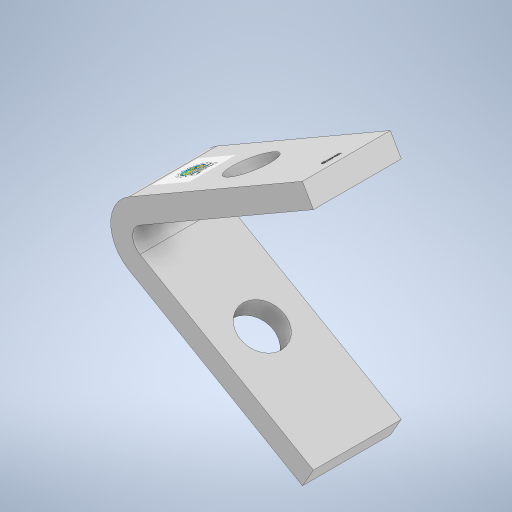
# Autodesk Inventor part: Part1
Saved by Autodesk Inventor 2023 (Build 270158000, 158)
## iProperties
Created: 2024-10-14
Part Number: Part1
Material: Generic
Document SubType Name: Modeling
Designer: students
Density: 1 g/cm^3
Appearance: Default
Author: students
Autodesk Inventor part; units mm, degrees
ref_plane "YZ Plane" through (0, 0, 0) normal (1, 0, 0) x (0, 1, 0)
ref_plane "XZ Plane" through (0, 0, 0) normal (0, 1, 0) x (-1, 0, 0)
ref_plane "XY Plane" through (0, 0, 0) normal (0, 0, 1) x (1, 0, 0)
sketch "Sketch1" plane through (0, 0, 0) normal (0, 0, 1) x (1, 0, 0)
  line L0 (57.8268, 26.3393) -> (176.2114, 94.6887)
  line L1 (20.3268, 4.6887) -> (157.0255, 4.6887) construction
  line L2 (57.8268, -16.9619) -> (176.2114, -85.3113)
  line L3 (20.3268, 4.6887) -> (157.0255, 4.6887) construction
  arc A0 (57.8268, 26.3393) -> (57.8268, -16.9619) centre (70.3268, 4.6887) ccw
  line L4 (183.7114, 81.6983) -> (65.3268, 13.3489)
  arc A1 (65.3268, 13.3489) -> (65.3268, -3.9716) centre (70.3268, 4.6887) ccw
  line L5 (65.3268, -3.9716) -> (183.7114, -72.3209)
  line L6 (176.2114, 94.6887) -> (183.7114, 81.6983)
  line L7 (183.7114, -72.3209) -> (176.2114, -85.3113)
  point P0 (0, 0)
  dimension "d0" = 180
  dimension "d2" = 180
  dimension "d4" = 25
  dimension "d5" = 15
  dimension "d7" = 60
  constraints: 16 end point, 4 point on circle, 2 centre point, 2 equal length, 2 horizontal, 2 point on line, 2 tangent, 2 other
  measures "d0" distance of L1.start L0.end
  measures "d2" distance of L1.start L2.end
  measures "d4" radius of A0
  measures "d5" distance between parallel lines of L0 L4
  measures "d7" angle of L5 L4
extrude "Extrusion1" add sketch "Sketch1" along normal blind 60
sketch "Sketch2" plane through (57.8268, 26.3393, 60) normal (-0.5, 0.8660254, 0) x (0.8660254, 0.5, 0)
  line L0 (136.6987, 60) -> (136.6987, 0) projected
  line L1 (136.6987, 60) -> (136.6987, 30)
  circle A0 centre (61.6987, 30) radius 15
  point P0 (-63.2492, 60)
  dimension "d10" = 30
  dimension "d12" = 30
  constraints: 2 end point, 1 centre point, 1 midpoint
  measures "d10" distance of L0.start L1.end
  measures "d12" diameter of A0
hole "Hole1" at (111.2595, 57.1887, 30) direction (0.5, -0.8660254, 0) diameter 30 depth 16 tip angle 118
sketch "Sketch3" plane through (176.2114, -85.3113, 0) normal (-0.5, -0.8660254, 0) x (0.8660254, -0.5, 0)
  line L0 (0, 60) -> (0, 30)
  line L1 (0, 0) -> (0, 60) projected
  line L2 (0, 30) -> (-75, 30)
  circle A0 centre (-75, 30) radius 15
  point P0 (-195.2592, 0)
  dimension "d20" = 30
  dimension "d21" = 75
  dimension "d22" = 30
  constraints: 4 end point, 1 centre point, 1 coincident, 1 midpoint, 1 perpendicular
  measures "d20" distance of L0.start L0.end
  measures "d21" distance of L0.end L2.end
  measures "d22" diameter of A0
hole "Hole2" at (111.2595, -47.8113, 30) direction (0.5, 0.8660254, 0) diameter 30 depth 16 tip angle 118
sketch "Sketch8" plane through (57.8268, 26.3393, 60) normal (-0.5, 0.8660254, 0) x (0.8660254, 0.5, 0)
  line L0 (124.5742, 21.8974) -> (124.5742, 35.2858) construction
  line L1 (124.5742, 35.2858) -> (128.6544, 35.2858) construction
  line L2 (128.6544, 35.2858) -> (128.6544, 21.8974) construction
  line L3 (128.6544, 21.8974) -> (124.5742, 21.8974) construction
  line L4 (0, 60) -> (0, 0) projected
  line L5 (0, 27.6079) -> (153.6173, 28.7907) construction
  line L6 (127.758, 23.9352) -> (127.758, 23.5499)
  line L7 (127.758, 23.5499) -> (127.5258, 23.5499)
  spline S0 degree 2 poles (127.5258, 23.5499) (127.5999, 23.461) (127.6987, 23.33) (127.7407, 23.2411) knots 0 0 0 1 2 2 2
  spline S1 degree 2 poles (127.7407, 23.2411) (127.7803, 23.1596) (127.8222, 22.9842) (127.8222, 22.8681) knots 0 0 0 1 2 2 2
  spline S2 degree 2 poles (127.8222, 22.8681) (127.8222, 22.6804) (127.6666, 22.3643) (127.516, 22.2531) knots 0 0 0 1 2 2 2
  spline S3 degree 2 poles (127.516, 22.2531) (127.3653, 22.142) (126.9207, 22.0185) (126.6317, 22.0185) knots 0 0 0 1 2 2 2
  spline S4 degree 2 poles (126.6317, 22.0185) (126.3304, 22.0185) (125.8907, 22.1741) (125.7252, 22.3099) knots 0 0 0 1 2 2 2
  spline S5 degree 2 poles (125.7252, 22.3099) (125.577, 22.4359) (125.4066, 22.7891) (125.4066, 22.9842) knots 0 0 0 1 2 2 2
  spline S6 degree 2 poles (125.4066, 22.9842) (125.4066, 23.1547) (125.4831, 23.4091) (125.5622, 23.5499) knots 0 0 0 1 2 2 2
  line L8 (125.5622, 23.5499) -> (124.5742, 23.5499)
  line L9 (124.5742, 23.5499) -> (124.5742, 23.9352)
  line L10 (124.5742, 23.9352) -> (127.758, 23.9352)
  line L11 (127.2023, 23.5499) -> (125.8808, 23.5499)
  spline S7 degree 2 poles (125.8808, 23.5499) (125.8117, 23.4066) (125.7598, 23.1794) (125.7598, 23.0485) knots 0 0 0 1 2 2 2
  spline S8 degree 2 poles (125.7598, 23.0485) (125.7598, 22.7521) (126.2044, 22.4161) (126.6243, 22.4161) knots 0 0 0 1 2 2 2
  spline S9 degree 2 poles (126.6243, 22.4161) (127.0294, 22.4161) (127.4567, 22.673) (127.4567, 22.9571) knots 0 0 0 1 2 2 2
  spline S10 degree 2 poles (127.4567, 22.9571) (127.4567, 23.1077) (127.3184, 23.414) (127.2023, 23.5499) knots 0 0 0 1 2 2 2
  line L12 (127.758, 26.2891) -> (127.758, 25.9038)
  line L13 (127.758, 25.9038) -> (126.4539, 25.9038)
  spline S11 degree 2 poles (126.4539, 25.9038) (126.2958, 25.9038) (126.0241, 25.8742) (125.9426, 25.8297) knots 0 0 0 1 2 2 2
  spline S12 degree 2 poles (125.9426, 25.8297) (125.8561, 25.7828) (125.7721, 25.6148) (125.7721, 25.4715) knots 0 0 0 1 2 2 2
  spline S13 degree 2 poles (125.7721, 25.4715) (125.7721, 25.3283) (125.9253, 25.0245) (126.0488, 24.8787) knots 0 0 0 1 2 2 2
  line L14 (126.0488, 24.8787) -> (127.758, 24.8787)
  line L15 (127.758, 24.8787) -> (127.758, 24.4934)
  line L16 (127.758, 24.4934) -> (124.5742, 24.4934)
  line L17 (124.5742, 24.4934) -> (124.5742, 24.8787)
  line L18 (124.5742, 24.8787) -> (125.7252, 24.8787)
  spline S14 degree 2 poles (125.7252, 24.8787) (125.5696, 25.0516) (125.4066, 25.3851) (125.4066, 25.5728) knots 0 0 0 1 2 2 2
  spline S15 degree 2 poles (125.4066, 25.5728) (125.4066, 25.9087) (125.8512, 26.2891) (126.2735, 26.2891) knots 0 0 0 1 2 2 2
  line L19 (126.2735, 26.2891) -> (127.758, 26.2891)
  spline S16 degree 2 poles (127.516, 28.1046) (127.5505, 28.0577) (127.674, 27.8996) (127.7111, 27.8255) knots 0 0 0 1 2 2 2
  spline S17 degree 2 poles (127.7111, 27.8255) (127.7654, 27.7242) (127.8222, 27.534) (127.8222, 27.3611) knots 0 0 0 1 2 2 2
  spline S18 degree 2 poles (127.8222, 27.3611) (127.8222, 27.2203) (127.716, 26.9659) (127.6197, 26.8696) knots 0 0 0 1 2 2 2
  spline S19 degree 2 poles (127.6197, 26.8696) (127.5258, 26.7782) (127.2492, 26.667) (127.0961, 26.667) knots 0 0 0 1 2 2 2
  spline S20 degree 2 poles (127.0961, 26.667) (126.8589, 26.667) (126.523, 26.8671) (126.4267, 27.0845) knots 0 0 0 1 2 2 2
  spline S21 degree 2 poles (126.4267, 27.0845) (126.3378, 27.2771) (126.2711, 27.8008) (126.2538, 28.1046) knots 0 0 0 1 2 2 2
  line L20 (126.2538, 28.1046) -> (126.1797, 28.1046)
  spline S22 degree 2 poles (126.1797, 28.1046) (126.0463, 28.1046) (125.8808, 28.0231) (125.8339, 27.949) knots 0 0 0 1 2 2 2
  spline S23 degree 2 poles (125.8339, 27.949) (125.787, 27.8749) (125.7573, 27.6624) (125.7573, 27.5488) knots 0 0 0 1 2 2 2
  spline S24 degree 2 poles (125.7573, 27.5488) (125.7573, 27.4154) (125.8364, 27.0548) (125.9129, 26.8745) knots 0 0 0 1 2 2 2
  line L21 (125.9129, 26.8745) -> (125.9129, 26.8523)
  line L22 (125.9129, 26.8523) -> (125.5202, 26.8523)
  spline S25 degree 2 poles (125.5202, 26.8523) (125.4905, 26.9585) (125.4164, 27.3562) (125.4164, 27.5513) knots 0 0 0 1 2 2 2
  spline S26 degree 2 poles (125.4164, 27.5513) (125.4164, 27.7884) (125.4905, 28.112) (125.5869, 28.2404) knots 0 0 0 1 2 2 2
  spline S27 degree 2 poles (125.5869, 28.2404) (125.6807, 28.3664) (125.9796, 28.4899) (126.1945, 28.4899) knots 0 0 0 1 2 2 2
  line L23 (126.1945, 28.4899) -> (127.758, 28.4899)
  line L24 (127.758, 28.4899) -> (127.758, 28.1046)
  line L25 (127.758, 28.1046) -> (127.516, 28.1046)
  line L26 (127.1949, 28.1046) -> (126.5601, 28.1046)
  spline S28 degree 2 poles (126.5601, 28.1046) (126.5724, 27.9663) (126.6144, 27.5488) (126.6539, 27.4179) knots 0 0 0 1 2 2 2
  spline S29 degree 2 poles (126.6539, 27.4179) (126.7009, 27.2648) (126.896, 27.0647) (127.0689, 27.0647) knots 0 0 0 1 2 2 2
  spline S30 degree 2 poles (127.0689, 27.0647) (127.2665, 27.0647) (127.4666, 27.287) (127.4666, 27.4994) knots 0 0 0 1 2 2 2
  spline S31 degree 2 poles (127.4666, 27.4994) (127.4666, 27.6797) (127.311, 27.9761) (127.1949, 28.1046) knots 0 0 0 1 2 2 2
  line L27 (125.8833, 30.2436) -> (125.8833, 30.2239)
  spline S32 degree 2 poles (125.8833, 30.2239) (125.8709, 30.1794) (125.866, 30.0831) (125.866, 30.0164) knots 0 0 0 1 2 2 2
  spline S33 degree 2 poles (125.866, 30.0164) (125.866, 29.8608) (126.0018, 29.5545) (126.1352, 29.4162) knots 0 0 0 1 2 2 2
  line L28 (126.1352, 29.4162) -> (127.758, 29.4162)
  line L29 (127.758, 29.4162) -> (127.758, 29.0308)
  line L30 (127.758, 29.0308) -> (125.4708, 29.0308)
  line L31 (125.4708, 29.0308) -> (125.4708, 29.4162)
  line L32 (125.4708, 29.4162) -> (125.8117, 29.4162)
  spline S34 degree 2 poles (125.8117, 29.4162) (125.6239, 29.6261) (125.4708, 29.9398) (125.4708, 30.088) knots 0 0 0 1 2 2 2
  spline S35 degree 2 poles (125.4708, 30.088) (125.4708, 30.1473) (125.4757, 30.2066) (125.4831, 30.2436) knots 0 0 0 1 2 2 2
  line L33 (125.4831, 30.2436) -> (125.8833, 30.2436)
  spline S36 degree 2 poles (127.8099, 31.5354) (127.8099, 30.9871) (127.1949, 30.3844) (126.6268, 30.3844) knots 0 0 0 1 2 2 2
  spline S37 degree 2 poles (126.6268, 30.3844) (126.0685, 30.3844) (125.4066, 30.9698) (125.4066, 31.4416) knots 0 0 0 1 2 2 2
  spline S38 degree 2 poles (125.4066, 31.4416) (125.4066, 31.654) (125.5301, 31.9825) (125.661, 32.1035) knots 0 0 0 1 2 2 2
  spline S39 degree 2 poles (125.661, 32.1035) (125.7919, 32.227) (126.1698, 32.3579) (126.444, 32.3579) knots 0 0 0 1 2 2 2
  line L34 (126.444, 32.3579) -> (126.6539, 32.3579)
  line L35 (126.6539, 32.3579) -> (126.6539, 30.7747)
  spline S40 degree 2 poles (126.6539, 30.7747) (127.0516, 30.7747) (127.474, 31.1748) (127.474, 31.5305) knots 0 0 0 1 2 2 2
  spline S41 degree 2 poles (127.474, 31.5305) (127.474, 31.6565) (127.4172, 31.901) (127.3727, 31.9998) knots 0 0 0 1 2 2 2
  spline S42 degree 2 poles (127.3727, 31.9998) (127.3233, 32.1035) (127.2369, 32.2468) (127.1973, 32.2937) knots 0 0 0 1 2 2 2
  line L36 (127.1973, 32.2937) -> (127.1973, 32.316)
  line L37 (127.1973, 32.316) -> (127.6172, 32.316)
  spline S43 degree 2 poles (127.6172, 32.316) (127.6444, 32.2493) (127.7234, 32.0467) (127.7457, 31.9677) knots 0 0 0 1 2 2 2
  spline S44 degree 2 poles (127.7457, 31.9677) (127.7778, 31.8565) (127.8099, 31.6738) (127.8099, 31.5354) knots 0 0 0 1 2 2 2
  spline S45 degree 2 poles (126.36, 31.9825) (126.2044, 31.9776) (125.9771, 31.9133) (125.9006, 31.8516) knots 0 0 0 1 2 2 2
  spline S46 degree 2 poles (125.9006, 31.8516) (125.8141, 31.7849) (125.7227, 31.575) (125.7227, 31.4193) knots 0 0 0 1 2 2 2
  spline S47 degree 2 poles (125.7227, 31.4193) (125.7227, 31.2662) (125.8141, 31.0513) (125.903, 30.9624) knots 0 0 0 1 2 2 2
  spline S48 degree 2 poles (125.903, 30.9624) (125.9944, 30.8759) (126.2143, 30.787) (126.36, 30.7747) knots 0 0 0 1 2 2 2
  line L38 (126.36, 30.7747) -> (126.36, 31.9825)
  line L39 (127.758, 34.5439) -> (127.758, 34.1586)
  line L40 (127.758, 34.1586) -> (126.4539, 34.1586)
  spline S49 degree 2 poles (126.4539, 34.1586) (126.2958, 34.1586) (126.0241, 34.129) (125.9426, 34.0845) knots 0 0 0 1 2 2 2
  spline S50 degree 2 poles (125.9426, 34.0845) (125.8561, 34.0376) (125.7721, 33.8696) (125.7721, 33.7263) knots 0 0 0 1 2 2 2
  spline S51 degree 2 poles (125.7721, 33.7263) (125.7721, 33.5831) (125.9253, 33.2793) (126.0488, 33.1335) knots 0 0 0 1 2 2 2
  line L41 (126.0488, 33.1335) -> (127.758, 33.1335)
  line L42 (127.758, 33.1335) -> (127.758, 32.7482)
  line L43 (127.758, 32.7482) -> (125.4708, 32.7482)
  line L44 (125.4708, 32.7482) -> (125.4708, 33.1335)
  line L45 (125.4708, 33.1335) -> (125.7252, 33.1335)
  spline S52 degree 2 poles (125.7252, 33.1335) (125.5696, 33.3064) (125.4066, 33.6399) (125.4066, 33.8276) knots 0 0 0 1 2 2 2
  spline S53 degree 2 poles (125.4066, 33.8276) (125.4066, 34.1635) (125.8512, 34.5439) (126.2735, 34.5439) knots 0 0 0 1 2 2 2
  line L46 (126.2735, 34.5439) -> (127.758, 34.5439)
  point P0 (-63.2492, 60)
  constraints: 2 end point, 1 point on line, 2 other
emboss "Emboss3" sketch "Sketch8" operation cut depth 1 direction (0.5, -0.8660254, 0)
sketch "Sketch9" plane through (57.8268, 26.3393, 60) normal (-0.5, 0.8660254, 0) x (0.8660254, 0.5, 0)
  line L0 (2.092, 45.4013) -> (36.0526, 45.4013) construction
  line L1 (36.0526, 45.4013) -> (36.0526, 13.4383) construction
  line L2 (36.0526, 13.4383) -> (2.092, 13.4383) construction
  line L3 (2.092, 13.4383) -> (2.092, 45.4013) construction
  point P0 (-63.2492, 60)
  constraints: 2 other
decal "Decal3"
body "Solid1"
